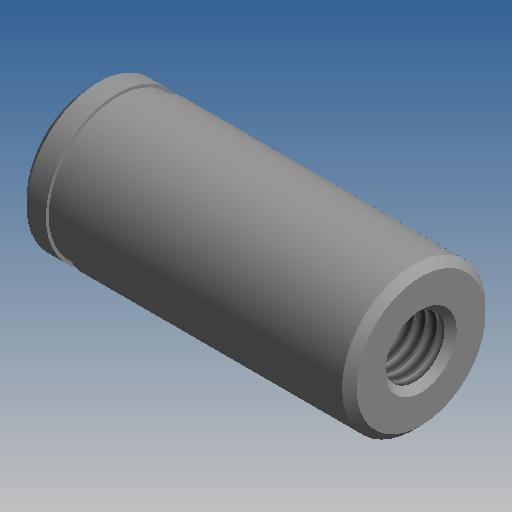
# Autodesk Inventor part: FSSFJBF-D10-L20-M5-U3
Saved by Autodesk Inventor 2020 (Build 240168000, 168)
## iProperties
Part Number: FSSFJBF-D10-L20-M5-U3
Material: 一般
Catalog Web Link: www.cadenas.de
Description: FSFJ_ _, FSSFJ_ _, FPSFJ_ _, FPSSFJ_ _, FSFU_ _, FSSFU_ _-Shafts - Shaft Ends Configurable
Vendor: MISUMI
Document SubType Name: Modeling
Designer: partserver
Manufacturer: MISUMI
Mass: 1.57965 g
Surface Area: 10.6928 cm^2
Volume: 1.57965 cm^3
Density: 1 g/cm^3
Appearance: PSOLRGB-175-175-175
Category: PARTsolutions
Company: MISUMI
PSOL_IDENT_0: {$CADENAS_DATA\23d-libs\misumi\metric\01_linear_shafts\fsfj.prj},385 {VTYP=3D},{NB=FSSFJBF-D10-L20-M
PSOL_IDENT_1: 5-U3},{LINA=FSSFJBF-D10-L20-M5-U3},{NN=FSFJ_ _, FSSFJ_ _, FPSFJ_ _, FPSSFJ_ _, FSFU_ _, FSSFU_ _},{D
PSOL_IDENT_2: ATE=06.07.2021 09:51:18},{GEOMDATE=14.05.2021 06:37:12},{VERSION=},{LINEID=10},{WBVAR=DTS,MAT,ST,LES
PSOL_IDENT_3: ,RES,D,ALT1,L,F,ALT9,M,PMC,PMS,B,T,ALT10,N,QMC,QMS,S,H,U,P,Q,R,W,J,Z,ALT3,SC,WSC,X},{WBNUMERIC=D,L,F
PSOL_IDENT_4: ,M,PMC,PMS,B,T,N,QMC,QMS,S,H,U,P,Q,R,W,J,Z,SC,WSC,X}  {NB=FSSFJBF-D10-L20-M5-U3},{LINA=FSSFJBF-D10-L
PSOL_IDENT_5: 20-M5-U3},{KT=DUMMY},{PN=FSSFJBF-D10-L20-M5-U3},{TYPE=FSSFJ},{TS=FSFJ_ _, FSSFJ_ _, FPSFJ_ _, FPSSFJ
PSOL_IDENT_6: _ _, FSFU_ _, FSSFU_ _},{DTS=g6},{DTSALG= 'g6','g6','h5','h5' },{MAT=SUS440C},{MATALG= 'SUJ2','52100
PSOL_IDENT_7: Bearing Steel','SUS440C','440C Stainless Steel Equivalent' },{ST=-},{STALG= '-','-','HCP','Hard Chr
PSOL_IDENT_8: ome Plating - Plating Hardness: HV750~ Plating Thickness: 5 micron or More' },{LES=B},{LESALG= 'A','
PSOL_IDENT_9: A','B','B','C','C','D','D','E','E','F','F','G','G','H','H','T','T' },{RES=F},{RESALG= 'A','A','B','B'
PSOL_IDENT_10: ,'C','C','D','D','E','E','F','F','G','G','H','H','T','T' },{CIFLESRES=1},{D=10},{DALG=[6:10/1],[12:2
PSOL_IDENT_11: 0/1],[22],[24:26/1],[28],[30],[32],[35],[40],[45],[50]},{ALT1=},{ALT1ALG= '','w/o LKC (L Dimension T
PSOL_IDENT_12: olerance Change)','LKC','with LKC (L Dimension Tolerance Change)' },{ALT1PN=},{L=20.0},{LALG=[20:497
PSOL_IDENT_13: /0.5]},{LMIN=20},{LMIN1=20},{LMIN2=0},{LMAX=497.0},{F=0.0},{FALG=[0:0/0.5]},{FMIN=0},{FMAX=0},{FPN=}
PSOL_IDENT_14: ,{CIFFMIN=1},{ALT9=},{ALT9ALG= '','N/A' },{ALT9PN=-M5},{CIFPMC1=1},{CIFPMC2=0},{CIFPMS1=1},{CIFPMS2=
PSOL_IDENT_15: 0},{M=5},{MALG=3,4,5},{MMIN=0},{MMAX=5},{BGMALG=3,4,5},{BMALG=3,4,5},{BMMAX=5},{BMMAX1=6},{BMMAX2=5}
PSOL_IDENT_16: ,{BMMAX3=0},{CMALG=3,4,5,6,8},{CMMIN=3},{CMMAX=8},{CMMAX1=10},{CMMAX2=8},{EGMALG=3,4,5,6},{EMALG=3,4
PSOL_IDENT_17: ,5,6},{EMMAX=6},{EMMAX1=6},{EMMAX2=20},{EMMAX3=0},{HGMALG=0},{HGMMAX=0},{HGMMAX1=5},{HGMMAX2=0},{HGM
PSOL_IDENT_18: MAX3=5},{HMALG=0},{HMMAX=1.5},{HMMAX1=1.5},{HMMAX2=5},{HMMAX3=0},{PMC=0},{PMCALG=0},{PMCMIN=0},{PMCM
PSOL_IDENT_19: IN1=0},{PMCMIN2=0},{PMCMAX=0},{PMCMAX1=10},{PMCMAX2=0},{PMS=0},{PMSALG=0},{PMSMIN=10},{PMSMIN1=10},{
PSOL_IDENT_20: PMSMIN2=10},{PMSMAX=0},{PMSMAX1=10},{PMSMAX2=0},{MPITCH=0.80},{PMCPITCH=0.00},{PMSPITCH=0.00},{ML=10
PSOL_IDENT_21: },{UM=16.5},{MIT=2},{MPN=-M5},{PM3D=0},{B=0},{BALG=[0]},{BMIN=3},{BMAX=-2},{BMAX1=-2},{BMAX2=15},{BM
PSOL_IDENT_22: AX3=0},{BPN=},{T=0.0},{TALG=[0:0/0.5]},{TMIN=0},{TMAX=0},{TPN=},{TMIN1=10},{ALT10=},{ALT10ALG= '','N
PSOL_IDENT_23: /A' },{ALT10PN=-N0},{CIFQMC1=1},{CIFQMC2=0},{CIFQMS1=1},{CIFQMS2=0},{N=0},{NALG=0},{CNALG=3,4,5,6,8}
PSOL_IDENT_24: ,{CNMIN=3},{CNMAX=8},{CNMAX1=10},{CNMAX2=8},{BBNALG=5},{BENALG=3,5},{BHNALG=0},{BHNMAX=0},{BHNMAX1=1
PSOL_IDENT_25: 2},{BHNMAX2=5},{BHNMAX3=0},{BHNMAX4=0},{EBNALG=5},{EENALG=5},{EHNMAX=0},{EHNMAX1=0},{EHNMAX2=5},{EHN
PSOL_IDENT_26: MAX3=0},{EHNALG=0},{GBNALG=3,4,5},{GENALG=3,4,5,6},{GHNALG=0},{GHNMAX=0},{GHNMAX1=5},{GHNMAX2=0},{GH
PSOL_IDENT_27: NMAX3=5},{HBNALG=0},{HBNMAX=0},{HBNMAX1=6},{HBNMAX2=0},{HBNMAX3=5},{HENALG=0},{HENMAX=0},{HENMAX1=6}
PSOL_IDENT_28: ,{HENMAX2=0},{HENMAX3=5},{HHNALG=0},{HHNMAX=0},{HHNMAX1=0},{HHNMAX2=0},{HHNMAX3=5},{OENALG=0},{OENMI
PSOL_IDENT_29: N=0},{OENMAX=0},{OENMAX1=5},{OENMAX2=0},{OEBNMAX=6},{OEENMAX=6},{OEHNMAX=0},{QMC=0},{QMCALG=0},{QMCM
PSOL_IDENT_30: IN=0},{QMCMIN1=0},{QMCMIN2=0},{QMCMAX=0},{QMCMAX1=10},{QMCMAX2=0},{QMS=0},{QMSALG=0},{QMSMIN=0},{QMS
PSOL_IDENT_31: MIN1=0},{QMSMIN2=0},{QMSMAX=0},{QMSMAX1=10},{QMSMAX2=0},{NPITCH=0.00},{QMCPITCH=0.00},{QMSPITCH=0.00
PSOL_IDENT_32: },{NL=0},{UN=0},{NIT=0},{NPN=},{QN3D=0},{S=0},{SALG=[0]},{SMIN=0},{SMIN1=0},{SMIN2=0},{SMAX=-2},{SMA
PSOL_IDENT_33: X1=-2},{SMAX2=0},{SMAX3=0},{SPN=},{H=0},{HALG=[0]},{HMIN=0},{HMAX=10},{HPN=},{U=3},{UALG=[3:10/1]},{
PSOL_IDENT_34: UMIN=3},{UMAX=10},{UPN=-U3},{MM=1.15},{DD=9.6},{P=0},{PALG=[0]},{PMIN=0},{DPMIN=0},{DPMIN1=4},{DPMIN
PSOL_IDENT_35: 2=0},{EPMIN=0},{EPMIN1=4},{EPMIN2=8},{EPMIN3=0},{EPMIN4=0},{PMAX=9},{PPN=},{Q=0},{QALG=[0]},{QMIN=0}
PSOL_IDENT_36: ,{QMIN1=4},{QMIN2=0},{EQMIN1=0},{EQMIN2=0},{QMAX=9},{QPN=},{R=0},{RALG=[0]},{RMIN=0},{RMAX=1},{RPN=}
PSOL_IDENT_37: ,{W=0},{WALG=[0]},{WMIN=0},{WMAX=6},{WPN=},{J=0},{JALG=[0]},{JMIN=0},{JMAX=0},{JMAX1=14},{JMAX2=0},{
PSOL_IDENT_38: JMAX3=14},{JPN=},{Z=0},{ZALG=[0]},{ZMIN=0},{ZMAX=0},{ZMAX1=14},{ZMAX2=0},{ZMAX3=14},{ZPN=},{BB=0.0},
PSOL_IDENT_39: {LL=0.0},{LSC=0.5},{LSEC=0.00},{RSC=0.5},{RSEC=0.00},{LSRR=0.0},{RSRR=0.0},{YMAX=500},{CIFMN=0},{CIF
PSOL_IDENT_40: MBB=0},{CIFNBB=0},{CIFGG=0},{ALT3=},{ALT3ALG= '','w/o Wrench Flats','SC','with SC (Wrench Flats at O
PSOL_IDENT_41: ne Location)','WSC','with WSC (Wrench Flats at Two Locations)' },{ALT3PN=},{SC=0},{SCALG=[0]},{SCMIN=
PSOL_IDENT_42: 0},{SCMAX=10},{WSC=0},{WSCALG=[0]},{WSCMIN=0},{WSCMAX=0},{X=0},{XALG=[0]},{XMIN=2},{XMAX=2},{CIFSC=0
PSOL_IDENT_43: },{CIFWSC=0},{CIFX=0},{LL1=0},{LL1ALG=8},{WALT3=0},{CIFBB=0},{ERRORPN=},{ERRORMALT3=OK},{ERRORNALT3=
PSOL_IDENT_44: OK},{ERRORLGALT3=OK},{ERRORRGALT3=OK},{FONTSIZE=1.000},{FSA=0.000}
NB: FSSFJBF-D10-L20-M5-U3
NN: FSFJ_ _, FSSFJ_ _, FPSFJ_ _, FPSSFJ_ _, FSFU_ _, FSSFU_ _
NT: Shafts - Shaft Ends Configurable
NBSYN: $PN.
LINA: FSSFJBF-D10-L20-M5-U3
CATALOG: Misumi
PN: FSSFJBF-D10-L20-M5-U3
TS: FSFJ_ _, FSSFJ_ _, FPSFJ_ _, FPSSFJ_ _, FSFU_ _, FSSFU_ _
DTS: g6
MAT: 440C Stainless Steel Equivalent
ST: -
LES: B
RES: F
D: 10
ALT1: w/o LKC (L Dimension Tolerance Change)
L: 20
F: 0
ALT9: N/A
M: 5
PMC: 0
PMS: 0
B: 0
T: 0
ALT10: N/A
N: 0
QMC: 0
QMS: 0
S: 0
H: 0
U: 3
MM: 1.15
DD: 9.6
P: 0
Q: 0
R: 0
W: 0
J: 0
Z: 0
BB: 0
LL: 0
LSC: 0.5
LSEC: 0
RSC: 0.5
RSEC: 0
LSRR: 0
RSRR: 0
ALT3: w/o Wrench Flats
SC: 0
WSC: 0
X: 0
LL1: 0
WALT3: 0
SUPPLIER: MISUMI
ARTICLENO: FSSFJBF-D10-L20-M5-U3
BOMINFO: FSSFJBF-D10-L20-M5-U3
CREATOR: CADENAS GmbH
Title: FSSFJBF-D10-L20-M5-U3
Author: Cadenas PARTsolutions
Comments: Shafts - Shaft Ends Configurable
Autodesk Inventor part; units mm, degrees
ref_plane "YZ Plane" through (0, 0, 0) normal (1, 0, 0) x (0, 1, 0)
ref_plane "XZ Plane" through (0, 0, 0) normal (0, 1, 0) x (-1, 0, 0)
ref_plane "XY Plane" through (0, 0, 0) normal (0, 0, 1) x (1, 0, 0)
sketch "Sketch_1" plane through (0, 0, 0) normal (0, 0, 1) x (1, 0, 0)
  line L0 (23, 0) -> (0, 0)
  line L1 (0, 0) -> (0, 4.5)
  line L2 (0, 4.5) -> (0.5, 5)
  line L3 (0.5, 5) -> (22.5, 5)
  line L4 (22.5, 5) -> (23, 4.5)
  line L5 (23, 4.5) -> (23, 0)
  line L6 (23, 0) -> (0, 0)
  constraints: 14 end point
revolve "Revolution1" add sketch "Sketch_1" angle 360 about axis through (23, 0, 0) along (1, 0, 0)
sketch "Sketch2" plane through (0, 0, 0) normal (-1, 0, 0) x (0, 0, 1)
  point P0 (0, 0)
hole "Hole1" at (0, 0, 0) direction (1, 0, 0) diameter 4.134 depth 15.3066 tip angle 120 countersink diameter 5 countersink angle 90 thread size "M5x0.8" class "6H" standard "ISO Metric profile"
sketch "Sketch_8" plane through (0, 0, 0) normal (0, 0, 1) x (1, 0, 0)
  line L0 (23, 0) -> (-23, 0)
  line L1 (20, 14.8) -> (20, 4.8)
  line L2 (20, 4.8) -> (21.15, 4.8)
  line L3 (21.15, 4.8) -> (21.15, 14.8)
  line L4 (21.15, 14.8) -> (20, 14.8)
  constraints: 10 end point
revolve "Revolution2" cut sketch "Sketch_8" angle 360 about axis through (23, 0, 0) along (1, 0, 0)
body "Solid1"
